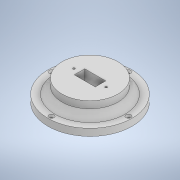
# Autodesk Inventor part: base 1
Saved by Autodesk Inventor 2022 (Build 260153000, 153)
## iProperties
Created: 2021-06-28
Part Number: base 1
Material: Generic
Document SubType Name: Modeling
Designer: USER
Density: 1 g/cm^3
Appearance: Default
Author: USER
Autodesk Inventor part; units mm, degrees
ref_plane "YZ Plane" through (0, 0, 0) normal (1, 0, 0) x (0, 1, 0)
ref_plane "XZ Plane" through (0, 0, 0) normal (0, 1, 0) x (-1, 0, 0)
ref_plane "XY Plane" through (0, 0, 0) normal (0, 0, 1) x (1, 0, 0)
sketch "Sketch1" plane through (0, 0, 0) normal (0, 1, 0) x (-1, 0, 0)
  circle A0 centre (0, 0) radius 55
  dimension "d0" = 110
  constraints: 1 centre point, 1 coincident
  measures "d0" diameter of A0
extrude "Extrusion1" add sketch "Sketch1" along normal blind 10
sketch "Sketch2" plane through (0, 10, 0) normal (0, 1, 0) x (1, 0, 0)
  circle A0 centre (0, 0) radius 50
  dimension "d3" = 100
  constraints: 1 centre point, 1 coincident
  measures "d3" diameter of A0
extrude "Extrusion2" add sketch "Sketch2" along normal blind 10
chamfer "Chamfer1" distance 10 angle 45 1 edges at (-50, 20, 0)
sketch "Sketch3" plane through (0, 20, 0) normal (0, 1, 0) x (1, 0, 0)
  circle A0 centre (0, 0) radius 40
  dimension "d9" = 80
  constraints: 1 centre point, 1 coincident
  measures "d9" diameter of A0
extrude "Extrusion3" add sketch "Sketch3" along normal blind 10
sketch "Sketch4" plane through (0, 10, 0) normal (0, 1, 0) x (1, 0, 0)
  circle A0 centre (0, 0) radius 60
  dimension "d12" = 120
  constraints: 1 centre point, 1 coincident
  measures "d12" diameter of A0
extrude "Extrusion4" add sketch "Sketch4" against normal blind 10
sketch "Sketch5" plane through (0, 10, 0) normal (0, 1, 0) x (1, 0, 0)
  circle A0 centre (0, 55) radius 3.625
  circle A1 centre (0, 0) radius 60 projected
  circle A2 centre (-55, 0) radius 3.625
  circle A3 centre (0, -55) radius 3.625
  circle A4 centre (55, 0) radius 3.625
  dimension "d15" = 7.25
  dimension "d16" = 55
  dimension "d19" = 360
  constraints: 4 centre point, 9 other
  measures "d15" diameter of A0
  measures "d16" distance of A1.centre A0.centre
extrude "Extrusion5" cut sketch "Sketch5" against normal blind 2.1735 draft -45 contours A0 | A2 | A3 | A4
sketch "Sketch6" plane through (0, 10, 0) normal (0, 1, 0) x (1, 0, 0)
  circle A0 centre (0, 55) radius 1.4515
  circle A1 centre (0, 0) radius 60 projected
  circle A2 centre (-55, 0) radius 1.4515
  circle A3 centre (0, -55) radius 1.4515
  circle A4 centre (55, 0) radius 1.4515
  dimension "d23" = 2.903
  dimension "d24" = 55
  dimension "d27" = 360
  constraints: 4 centre point, 9 other
  measures "d23" diameter of A0
  measures "d24" distance of A1.centre A0.centre
extrude "Extrusion6" cut sketch "Sketch6" against normal through all contours A0 | A2 | A3 | A4
sketch "Sketch7" plane through (0, 30, 0) normal (0, 1, 0) x (1, 0, 0)
  line L0 (15, 7.5) -> (-15, 7.5)
  line L1 (-15, 7.5) -> (-15, -7.5)
  line L2 (-15, -7.5) -> (15, -7.5)
  line L3 (15, -7.5) -> (15, 7.5)
  line L4 (15, 7.5) -> (-15, -7.5) construction
  line L5 (-15, 7.5) -> (15, -7.5) construction
  point P0 (0, 0)
  dimension "d31" = 30
  dimension "d32" = 15
  constraints: 12 end point, 2 midpoint, 2 parallel, 1 horizontal, 1 perpendicular
  measures "d31" distance of L2.end L1.end
  measures "d32" distance of L1.end L0.end
extrude "Extrusion7" cut sketch "Sketch7" against normal through all
sketch "Sketch8" plane through (0, 30, 0) normal (0, 1, 0) x (1, 0, 0)
  circle A0 centre (-23, 0) radius 1.4515
  circle A1 centre (0, 0) radius 40 projected
  circle A2 centre (23, 0) radius 1.4515
  dimension "d35" = 2.903
  dimension "d36" = 23
  dimension "d39" = 360
  constraints: 2 centre point, 5 other
  measures "d35" diameter of A0
  measures "d36" distance of A1.centre A0.centre
extrude "Extrusion8" cut sketch "Sketch8" against normal through all contours A0 | A2
body "Solid1"
